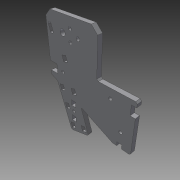
# Autodesk Inventor part: z_axis_top
Saved by Autodesk Inventor 2014 (Build 180170000, 170)
## iProperties
Created: 2014-03-30
Part Number: z_axis_top
Material: Plywood, Finish
Document SubType Name: Modeling
Designer: buben
Density: 0.552 g/cm^3
Appearance: Plywood - New
Author: buben
Autodesk Inventor part; units mm, degrees
ref_plane "YZ Plane" through (0, 0, 0) normal (1, 0, 0) x (0, 1, 0)
ref_plane "XZ Plane" through (0, 0, 0) normal (0, 1, 0) x (-1, 0, 0)
ref_plane "XY Plane" through (0, 0, 0) normal (0, 0, 1) x (1, 0, 0)
sketch "Sketch1" plane through (0, 0, 0) normal (0, 1, 0) x (-1, 0, 0)
  line L0 (0, -6) -> (0, 0)
  line L1 (0, 0) -> (-12, 0)
  line L2 (-12, 0) -> (-12, 13)
  line L3 (-12, 13) -> (0, 13)
  line L4 (0, 13) -> (0, 67)
  line L5 (0, 67) -> (-8, 75)
  line L6 (-8, 75) -> (-67, 75)
  line L7 (-67, 75) -> (-75, 67)
  line L8 (0, -6) -> (-100, -50)
  line L9 (-100, -50) -> (-124.5, -50)
  line L10 (-124.5, -50) -> (-124.5, 0)
  line L11 (-124.5, 0) -> (-118.5, 0)
  line L12 (-118.5, 0) -> (-118.5, 13)
  line L13 (-118.5, 13) -> (-124.5, 13)
  line L14 (-124.5, 13) -> (-124.5, 19)
  line L15 (-124.5, 19) -> (-75, 19)
  line L16 (-75, 19) -> (-75, 67)
  circle A0 centre (-26, 55) radius 4
  circle A1 centre (-49, 55) radius 2.5
  line L17 (-106, -50) -> (-112.5, -50) construction
  line L18 (-112.5, -50) -> (-112.5, 13) construction
  line L19 (-112.5, 13) -> (-106, 13) construction
  line L20 (-106, 13) -> (-106, -50) construction
  dimension "d0" = 13
  dimension "d1" = 12
  dimension "d2" = 6
  dimension "d3" = 6
  dimension "d4" = 6
  dimension "d6" = 75
  dimension "d7" = 8
  dimension "d8" = 5
  dimension "d9" = 23
  dimension "d10" = 106.5
  dimension "d11" = 45
  dimension "d12" = 8
  dimension "d13" = 6.5
  dimension "d14" = 6
  dimension "d15" = 6
  dimension "d16" = 42
  dimension "d17" = 20
  dimension "d18" = 50
  dimension "d19" = 26
  constraints: 42 end point, 10 perpendicular, 7 collinear, 7 parallel, 2 centre point, 1 horizontal, 1 horizontal alignment, 1 vertical
  measures "d0" distance of L1.end L2.end
  measures "d1" distance of L0.end L1.end
  measures "d2" distance of L10.end L11.end
  measures "d3" distance of L0.start L0.end
  measures "d4" distance of L13.end L14.end
  measures "d6" distance between parallel lines of L16 L4
  measures "d7" diameter of A0
  measures "d8" diameter of A1
  measures "d9" distance of A1.centre A0.centre
  measures "d10" distance between parallel lines of L2 L12
  measures "d11" angle of L4 L5
  measures "d12" horizontal distance of L4.end L5.end
  measures "d13" distance of L18.end L19.end
  measures "d14" distance between parallel lines of L12 L18
  measures "d15" distance from line of L8.end L20
  measures "d16" distance from line of L3 A0.centre
  measures "d17" distance from line of L6 A0.centre
  measures "d18" distance between parallel lines of L9 L11
  measures "d19" distance from line of L4 A0.centre
extrude "Extrusion1" add sketch "Sketch1" along normal blind 6.5
sketch "Sketch3" plane through (0, 6.5, 0) normal (0, 1, 0) x (1, 0, 0)
  line L0 (124.5, 0) -> (124.5, 50) projected
  line L1 (124.5, 50) -> (100, 50) projected
  line L2 (106, 50) -> (112.5, 50)
  line L3 (112.5, 50) -> (112.5, 44)
  line L4 (112.5, 44) -> (106, 44)
  line L5 (106, 44) -> (106, 50)
  dimension "d27" = 6
  dimension "d28" = 6.5
  dimension "d29" = 12
  constraints: 8 end point, 2 parallel, 1 horizontal, 1 perpendicular, 1 point on line
  measures "d27" distance of L4.end L2.start
  measures "d28" distance of L3.end L4.end
  measures "d29" distance between parallel lines of L0 L3
extrude "Extrusion3" cut sketch "Sketch3" against normal through all
chamfer "Chamfer1" distance 2 angle 45 3 edges at (75, 3.25, 19) (124.5, 3.25, 19) (124.5, 3.25, -50)
sketch "Sketch4" plane through (0, 6.5, 0) normal (0, 1, 0) x (1, 0, 0)
  line L0 (124.5, 0) -> (124.5, 48) projected
  circle A0 centre (26, -55) radius 4 projected
  circle A1 centre (49, -55) radius 2.5 projected
  circle A2 centre (37.5, -47.5) radius 2.25
  circle A3 centre (37.5, -62.5) radius 2.25
  line L1 (37.5, -47.5) -> (37.5, -62.5) construction
  line L2 (26, -55) -> (49, -55) construction
  point P0 (37.5, -55)
  dimension "d35" = 15
  dimension "d36" = 4.5
  constraints: 4 end point, 2 centre point, 2 midpoint, 1 equal radius, 1 parallel, 1 perpendicular, 1 vertical alignment
  measures "d35" distance of L1.end L1.start
  measures "d36" diameter of A2
extrude "Extrusion4" cut sketch "Sketch4" against normal through all contours A2 | A3
sketch "Sketch5" plane through (0, 6.5, 0) normal (0, 1, 0) x (1, 0, 0)
  line L0 (106, 44) -> (106, 50) projected
  line L1 (100, 50) -> (0, 6) projected
  line L2 (0, 6) -> (0, 0) projected
  line L3 (0, 0) -> (12, 0) projected
  line L4 (12, -13) -> (0, -13) projected
  line L5 (0, -13) -> (0, -67) projected
  line L6 (53, 88) -> (6.5, -55) construction
  line L7 (10.7922, 10.7486) -> (32.0112, 76.0025)
  line L8 (32.0112, 76.0025) -> (62.9182, 65.9523)
  line L9 (62.9182, 65.9523) -> (50.6734, 28.2963)
  line L10 (50.6734, 28.2963) -> (10.7922, 10.7486)
  circle A0 centre (6.5, -55) radius 0.9 construction
  circle A1 centre (53, 88) radius 0.9 construction
  point P0 (47.4647, 70.9774)
  dimension "d39" = 42
  dimension "d40" = 6.5
  dimension "d41" = 106
  dimension "d42" = 53
  dimension "d43" = 88
  dimension "d44" = 32.5
  dimension "d45" = 1.8
  dimension "d46" = 17.9
  constraints: 10 end point, 3 point on line, 2 centre point, 2 coincident, 2 parallel, 1 collinear, 1 equal radius, 1 midpoint, 1 perpendicular
  measures "d39" distance from line of L6.end L4
  measures "d40" distance from line of L6.end L5
  measures "d41" distance between parallel lines of L2 L0
  measures "d42" distance from line of L6.start L2
  measures "d43" distance from line of L6.start L3
  measures "d44" distance between parallel lines of L9 L7
  measures "d45" diameter of A1
  measures "d46" distance from line of L6.start L8
extrude "Extrusion5" add sketch "Sketch5" against normal blind 6.5
sketch "Sketch6" plane through (0, 6.5, 0) normal (0, 1, 0) x (1, 0, 0)
  line L0 (50.6734, 28.2963) -> (62.9182, 65.9523) projected
  line L1 (62.9182, 65.9523) -> (32.0112, 76.0025) projected
  line L2 (32.0112, 76.0025) -> (10.7922, 10.7486) projected
  line L3 (33.6272, 71.2708) -> (39.8086, 69.2608)
  line L4 (39.8086, 69.2608) -> (37.3347, 61.6529)
  line L5 (37.3347, 61.6529) -> (31.1533, 63.6629)
  line L6 (31.1533, 63.6629) -> (33.6272, 71.2708)
  line L7 (52.6469, 65.0861) -> (58.8283, 63.076)
  line L8 (58.8283, 63.076) -> (56.3544, 55.4682)
  line L9 (56.3544, 55.4682) -> (50.173, 57.4782)
  line L10 (50.173, 57.4782) -> (52.6469, 65.0861)
  line L11 (17.2376, 20.8686) -> (23.419, 18.8586)
  line L12 (23.419, 18.8586) -> (20.9451, 11.2507)
  line L13 (20.9451, 11.2507) -> (14.7637, 13.2607)
  line L14 (14.7637, 13.2607) -> (17.2376, 20.8686)
  line L15 (24.8156, -20.5026) -> (30.997, -22.5126)
  line L16 (30.997, -22.5126) -> (28.5231, -30.1205)
  line L17 (28.5231, -30.1205) -> (22.3417, -28.1105)
  line L18 (22.3417, -28.1105) -> (24.8156, -20.5026)
  line L19 (24.9685, 44.6432) -> (31.15, 42.6332)
  line L20 (31.15, 42.6332) -> (28.6761, 35.0253)
  line L21 (28.6761, 35.0253) -> (22.4947, 37.0353)
  line L22 (22.4947, 37.0353) -> (24.9685, 44.6432)
  line L23 (37.185, 17.5368) -> (43.3665, 15.5268)
  line L24 (43.3665, 15.5268) -> (40.8926, 7.9189)
  line L25 (40.8926, 7.9189) -> (34.7112, 9.9289)
  line L26 (34.7112, 9.9289) -> (37.185, 17.5368)
  dimension "d49" = 6.5
  dimension "d50" = 3
  dimension "d52" = 3
  dimension "d53" = 4
  dimension "d54" = 8
  dimension "d57" = 45
  dimension "d58" = 20
  dimension "d59" = 82
  dimension "d60" = 42
  constraints: 48 end point, 12 parallel, 8 collinear, 8 perpendicular, 7 equal length
  measures "d49" distance of L3.start L3.end
  measures "d50" distance between parallel lines of L2 L6
  measures "d52" distance between parallel lines of L0 L8
  measures "d53" distance between parallel lines of L1 L3
  measures "d54" distance of L3.end L4.end
  measures "d57" distance between parallel lines of L5 L11
  measures "d58" distance between parallel lines of L5 L19
  measures "d59" distance between parallel lines of L15 L9
  measures "d60" distance between parallel lines of L9 L23
extrude "Extrusion6" cut sketch "Sketch6" against normal through all
sketch "Sketch7" plane through (0, 6.5, 0) normal (0, 1, 0) x (1, 0, 0)
  line L0 (32.0112, 76.0025) -> (10.7922, 10.7486) projected
  line L1 (12, -13) -> (0, -13) projected
  line L2 (0, -13) -> (0, -67) projected
  line L3 (5.2631, -58.8039) -> (7.7369, -51.1961) construction
  line L4 (2.8856, -58.0308) -> (5.3595, -50.423)
  line L5 (10.1144, -51.9692) -> (7.6405, -59.577)
  arc A0 (2.8856, -58.0308) -> (7.6405, -59.577) centre (5.2631, -58.8039) ccw
  arc A1 (10.1144, -51.9692) -> (5.3595, -50.423) centre (7.7369, -51.1961) ccw
  point P0 (6.5, -55)
  point P1 (6.5, -55)
  dimension "d63" = 42
  dimension "d64" = 6.5
  dimension "d65" = 5
  dimension "d66" = 8
  constraints: 8 end point, 4 point on circle, 4 tangent, 2 centre point, 2 parallel, 1 coincident, 1 midpoint
  measures "d63" distance from line of point (6.5, -55) L1
  measures "d64" distance from line of L2 point (6.5, -55)
  measures "d65" distance between parallel lines of L5 L4
  measures "d66" distance of L3.start L3.end
extrude "Extrusion7" cut sketch "Sketch7" against normal through all
chamfer "Chamfer2" distance 2 angle 45 3 edges at (32.0112, 3.25, -76.0025) (62.9182, 3.25, -65.9523) (50.6734, 3.25, -28.2963)
sketch "Sketch8" plane through (0, 6.5, 0) normal (0, 1, 0) x (1, 0, 0)
  line L0 (12, 0) -> (12, -13) projected
  line L1 (0, -13) -> (0, -67) projected
  circle A0 centre (22.217, -6.5) radius 2.25
  point P0 (12, -6.5)
  dimension "d72" = 4.5
  dimension "d73" = 22.217
  constraints: 1 centre point, 1 horizontal alignment, 1 midpoint
  measures "d72" diameter of A0
  measures "d73" distance from line of L1 A0.centre
extrude "Extrusion8" cut sketch "Sketch8" against normal through all
sketch "Sketch9" plane through (0, 6.5, 0) normal (0, 1, 0) x (1, 0, 0)
  line L0 (0, 6) -> (0, 0) projected
  line L1 (0, 0) -> (12, 0) projected
  line L2 (34.828, 57.5) -> (41.328, 57.5)
  line L3 (41.328, 57.5) -> (41.328, 49.5)
  line L4 (41.328, 49.5) -> (34.828, 49.5)
  line L5 (34.828, 49.5) -> (34.828, 57.5)
  line L6 (34.828, 34.5) -> (41.328, 34.5)
  line L7 (41.328, 34.5) -> (41.328, 26.5)
  line L8 (41.328, 26.5) -> (34.828, 26.5)
  line L9 (34.828, 26.5) -> (34.828, 34.5)
  circle A0 centre (38.078, 42) radius 2.25
  point P0 (38.078, 49.5)
  dimension "d76" = 8
  dimension "d77" = 6.5
  dimension "d78" = 15
  dimension "d79" = 4.5
  dimension "d80" = 7.5
  dimension "d81" = 38.078
  dimension "d82" = 42
  constraints: 16 end point, 4 parallel, 3 collinear, 2 horizontal, 2 perpendicular, 1 centre point, 1 midpoint, 1 vertical alignment
  measures "d76" distance of L4.end L2.start
  measures "d77" distance of L2.start L2.end
  measures "d78" distance between parallel lines of L6 L4
  measures "d79" diameter of A0
  measures "d80" distance of point (38.078, 49.5) A0.centre
  measures "d81" distance from line of L0 A0.centre
  measures "d82" distance from line of L1 A0.centre
extrude "Extrusion9" cut sketch "Sketch9" against normal through all
sketch "Sketch10" plane through (0, 6.5, 0) normal (0, 1, 0) x (1, 0, 0)
  circle A0 centre (22.217, -6.5) radius 2.25 projected
  line L0 (118.5, -13) -> (118.5, 0) projected
  line L1 (118.5, 0) -> (124.5, 0) projected
  line L2 (112.5, 44) -> (106, 44) projected
  circle A1 centre (93.5, -6.5) radius 2.25
  circle A2 centre (109.25, 28) radius 2.25
  point P0 (109.25, 44)
  dimension "d85" = 25
  dimension "d86" = 28
  constraints: 2 centre point, 2 equal radius, 1 horizontal alignment, 1 midpoint, 1 vertical alignment
  measures "d85" distance from line of L0 A1.centre
  measures "d86" distance from line of L1 A2.centre
extrude "Extrusion10" cut sketch "Sketch10" against normal through all contours A1 | A2
equation "\"d2\" = d3"
equation "\"d4\" = d3"
equation "\"d42\" = 0.5 * d41"
equation "\"d80\" = 0.5 * d78"
body "Solid1"
